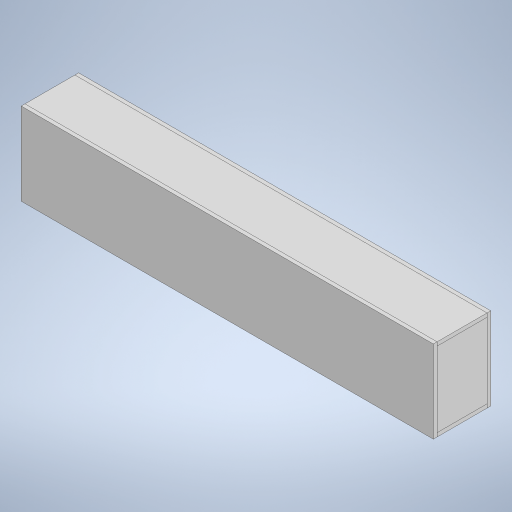
# Autodesk Inventor part: 0.75 box for battery pack
Saved by Autodesk Inventor 2024 (Build 280153020, 153B)
## iProperties
Created: 2023-08-06
Part Number: 0.75 box for battery pack
Material: Generic
Document SubType Name: Modeling
Designer: torban
Density: 1 g/cm^3
Appearance: Default
Author: torban
Autodesk Inventor part; units mm, degrees
ref_plane "YZ Plane" through (0, 0, 0) normal (1, 0, 0) x (0, 1, 0)
ref_plane "XZ Plane" through (0, 0, 0) normal (0, 1, 0) x (-1, 0, 0)
ref_plane "XY Plane" through (0, 0, 0) normal (0, 0, 1) x (1, 0, 0)
sketch "Sketch1" plane through (0, 0, 0) normal (0, 1, 0) x (-1, 0, 0)
  line L0 (0, 0) -> (2057.4, 0)
  line L1 (2057.4, 0) -> (2057.4, -254)
  line L2 (2057.4, -254) -> (0, -254)
  line L3 (0, -254) -> (0, 0)
  dimension "d0" = 2057.4
  dimension "d1" = 254
  constraints: 8 end point, 2 parallel, 1 horizontal, 1 perpendicular
  measures "d0" distance of L1.end L2.end
  measures "d1" distance of L0.end L1.end
extrude "Extrusion1" add sketch "Sketch1" along normal blind 381
sketch "Sketch2" plane through (0, 0, 0) normal (0, -1, 0) x (1, 0, 0)
  line L0 (0, 0) -> (0, -254) projected
  line L1 (0, -254) -> (-2057.4, -254) projected
  line L2 (-2057.4, -254) -> (-2057.4, 0) projected
  line L3 (-2057.4, 0) -> (0, 0) projected
  line L4 (-2057.4, 0) -> (0, 0) projected
  line L5 (0, 0) -> (19.05, 0)
  line L6 (19.05, 0) -> (19.05, -254)
  line L7 (19.05, -254) -> (0, -254)
  line L8 (0, -254) -> (0, 0)
  line L9 (-2057.4, 0) -> (-2076.45, 0)
  line L10 (-2076.45, 0) -> (-2076.45, -254)
  line L11 (-2076.45, -254) -> (-2057.4, -254)
  line L12 (-2057.4, -254) -> (-2057.4, 0)
  dimension "d4" = 19.05
  dimension "d5" = 19.05
  dimension "d6" = 0
  constraints: 16 end point, 4 parallel, 2 horizontal, 2 perpendicular, 1 point on line
  measures "d4" distance of L6.end L7.end
  measures "d5" distance of L11.end L10.end
  measures "d6" distance between parallel lines of L1 L7
extrude "Extrusion2" add sketch "Sketch2" along normal blind 19.05 separate body
sketch "Sketch3" plane through (0, 0, 0) normal (0, 1, 0) x (1, 0, 0)
  line L0 (0, 254) -> (0, 0) projected
  line L1 (0, 0) -> (-2057.4, 0) projected
  line L2 (-2057.4, 0) -> (-2057.4, 254) projected
  line L3 (-2057.4, 254) -> (0, 254) projected
  line L4 (19.05, 0) -> (-2076.45, 0) projected
  line L5 (-2076.45, 0) -> (-2076.45, 254) projected
  line L6 (-2076.45, 254) -> (19.05, 254) projected
  line L7 (19.05, 254) -> (19.05, 0) projected
extrude "Extrusion3" add sketch "Sketch3" along normal up to surface (381 mm away) separate body contours L6 L7 L4 L0 | L2 L4 L5 L6
sketch "Sketch4" plane through (0, 381, 0) normal (0, 1, 0) x (1, 0, 0)
  line L0 (0, 254) -> (0, 0) projected
  line L1 (0, 0) -> (-2057.4, 0) projected
  line L2 (-2057.4, 0) -> (-2057.4, 254) projected
  line L3 (-2057.4, 254) -> (0, 254) projected
  line L4 (-2057.4, 254) -> (-2057.4, 0) projected
  line L5 (-2057.4, 0) -> (-2076.45, 0) projected
  line L6 (-2076.45, 0) -> (-2076.45, 254) projected
  line L7 (-2076.45, 254) -> (-2057.4, 254) projected
  line L8 (19.05, 254) -> (19.05, 0) projected
  line L9 (19.05, 0) -> (0, 0) projected
  line L10 (0, 0) -> (0, 254) projected
  line L11 (0, 254) -> (19.05, 254) projected
extrude "Extrusion4" add sketch "Sketch4" along normal blind 19.05 separate body
sketch "Sketch5" plane through (-2057.4, 0, 0) normal (0, 0, 1) x (1, 0, 0)
  line L0 (2057.4, 381) -> (2057.4, 0) projected
  line L1 (2057.4, 0) -> (0, 0) projected
  line L2 (0, 0) -> (0, 381) projected
  line L3 (0, 381) -> (2057.4, 381) projected
  line L4 (-19.05, 0) -> (2076.45, 0) projected
  line L5 (2076.45, 0) -> (2076.45, -19.05) projected
  line L6 (2076.45, -19.05) -> (-19.05, -19.05) projected
  line L7 (-19.05, -19.05) -> (-19.05, 0) projected
  line L8 (0, 381) -> (0, 0) projected
  line L9 (0, 0) -> (-19.05, 0) projected
  line L10 (-19.05, 0) -> (-19.05, 381) projected
  line L11 (-19.05, 381) -> (0, 381) projected
  line L12 (2076.45, 0) -> (2057.4, 0) projected
  line L13 (2057.4, 0) -> (2057.4, 381) projected
  line L14 (2057.4, 381) -> (2076.45, 381) projected
  line L15 (2076.45, 381) -> (2076.45, 0) projected
  line L16 (2076.45, 400.05) -> (2076.45, 381) projected
  line L17 (2076.45, 381) -> (-19.05, 381) projected
  line L18 (-19.05, 381) -> (-19.05, 400.05) projected
  line L19 (-19.05, 400.05) -> (2076.45, 400.05) projected
extrude "Extrusion5" add sketch "Sketch5" along normal blind 19.05 separate body
sketch "Sketch6" plane through (0, 0, -254) normal (0, 0, -1) x (-1, 0, 0)
  line L0 (2057.4, 381) -> (2057.4, 0) projected
  line L1 (2057.4, 0) -> (0, 0) projected
  line L2 (0, 0) -> (0, 381) projected
  line L3 (0, 381) -> (2057.4, 381) projected
  line L4 (-19.05, -19.05) -> (-19.05, 0) projected
  line L5 (-19.05, 0) -> (2076.45, 0) projected
  line L6 (2076.45, 0) -> (2076.45, -19.05) projected
  line L7 (2076.45, -19.05) -> (-19.05, -19.05) projected
  line L8 (2076.45, 381) -> (2076.45, 0) projected
  line L9 (2076.45, 0) -> (2057.4, 0) projected
  line L10 (2057.4, 0) -> (2057.4, 381) projected
  line L11 (2057.4, 381) -> (2076.45, 381) projected
  line L12 (0, 0) -> (-19.05, 0) projected
  line L13 (-19.05, 0) -> (-19.05, 381) projected
  line L14 (-19.05, 381) -> (0, 381) projected
  line L15 (0, 381) -> (0, 0) projected
  line L16 (2076.45, 381) -> (-19.05, 381) projected
  line L17 (-19.05, 381) -> (-19.05, 400.05) projected
  line L18 (-19.05, 400.05) -> (2076.45, 400.05) projected
  line L19 (2076.45, 400.05) -> (2076.45, 381) projected
extrude "Extrusion6" add sketch "Sketch6" along normal blind 19.05 separate body
body "Solid1"
body "Solid4"
